Autodesk Fusion 360 part; units mm, degrees
(part 6 of 6)
sketch "Sketch25" plane through (0, 0, 0) normal (0, 1, 0) x (1, 0, 0)
  line L0 (85, 25) -> (135, 25)
  line L1 (135, 25) -> (135, -80)
  line L2 (135, -80) -> (85, -80)
  line L3 (85, -80) -> (85, 25)
  constraint horizontal L0
  constraint vertical L1
  constraint horizontal L2
  constraint vertical L3
extrude "Extrude24" add sketch "Sketch25" along normal blind 75 separate body makes body 16
sketch "Sketch26" plane through (135, 0, 0) normal (1, 0, 0) x (0, 0, -1)
  line L0 (-80, 0) -> (25, 0)
  line L1 (25, 0) -> (25, 75)
  line L2 (25, 75) -> (-80, 75)
  line L3 (-80, 75) -> (-80, 0)
  line L4 (-79, 3) -> (24, 3)
  circle A0 centre (-27.5, 3) radius 48
  line L5 (-80, 58) -> (25, 58)
  line L6 (-27.5, 58) -> (-27.5, 51)
  constraint perpendicular L1 L4
  constraint coincident L4 A0.centre
  constraint coincident L1 L5.end
  constraint perpendicular L1 L5
  constraint midpoint L5 L6.start
  constraint coincident A0 L6.end
  constraint perpendicular L5 L6
extrude "Extrude25" cut sketch "Sketch26" against normal blind 52 contours L0 L3 A0 L5 L6 | L1 L2 L3 L5 | L4 A0 bodies 16
sketch "Sketch27" plane through (135, 0, 0) normal (1, 0, 0) x (0, 0, -1)
  arc A0 (-75.5, 3) -> (-75.4062, 0) centre (-27.5, 3) ccw
  line L0 (-75.4062, 0) -> (25, 0)
  line L1 (25, 0) -> (25, 58)
  line L2 (25, 58) -> (-27.5, 58)
  line L3 (-27.5, 58) -> (-27.5, 51)
  arc A1 (20.5, 3) -> (-27.5, 51) centre (-27.5, 3) ccw
  line L4 (20.5, 3) -> (-75.5, 3)
  circle A2 centre (-27.5, 3) radius 52.5
  constraint concentric A0 A2
  constraint tangent L1 A2
extrude "Extrude26" cut sketch "Sketch27" against normal blind 52 contours L1 L2 L3 A2 bodies 16
hidden bodies 1 13 14 15 16
